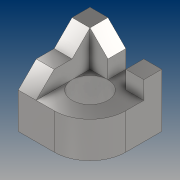
# Autodesk Inventor part: 20
Saved by Autodesk Inventor 2020.2 (Build 242310000, 310)
## iProperties
Created: 2020-09-17
Part Number: 20
Material: 鋼、碳鋼
Document SubType Name: Modeling
Designer: user
Density: 7.85 g/cm^3
Appearance: 半拋光
Mass: 247.275 g
Surface Area: 86.0922 cm^2
Volume: 31.5 cm^3
Author: user
Autodesk Inventor part; units mm, degrees
ref_plane "YZ Plane" through (0, 0, 0) normal (1, 0, 0) x (0, 1, 0)
ref_plane "XZ Plane" through (0, 0, 0) normal (0, 1, 0) x (-1, 0, 0)
ref_plane "XY Plane" through (0, 0, 0) normal (0, 0, 1) x (1, 0, 0)
sketch "草圖1" plane through (0, 0, 0) normal (0, 1, 0) x (-1, 0, 0)
  line L0 (0, 0) -> (-40, 0)
  line L1 (-40, 0) -> (-40, 20)
  arc A0 (-20, 40) -> (-40, 20) centre (-20, 20) ccw
  line L2 (-20, 40) -> (0, 40)
  line L3 (0, 40) -> (0, 0)
  dimension "d0" = 40
  dimension "d1" = 40
  dimension "d2" = 20
  constraints: 8 end point, 3 perpendicular, 2 point on circle, 2 tangent, 1 centre point, 1 horizontal
  measures "d0" distance of L0.start L0.end
  measures "d1" distance of L2.end L0.start
  measures "d2" distance of L2.start L2.end
extrude "擠出1" add sketch "草圖1" along normal blind 20
sketch "草圖2" plane through (0, 0, 0) normal (-1, 0, 0) x (0, 0, 1)
  line L0 (0, 0) -> (0, 20) projected
  line L1 (0, 20) -> (40, 20) projected
  line L2 (40, 20) -> (40, 0) projected
  line L3 (40, 0) -> (0, 0) projected
  line L4 (40, 20) -> (30, 30)
  line L5 (30, 30) -> (20, 30)
  line L6 (20, 30) -> (10, 40)
  line L7 (10, 40) -> (0, 40)
  line L8 (0, 40) -> (0, 20)
  line L9 (40, 20) -> (0, 20)
  dimension "d5" = 10
  dimension "d6" = 10
  dimension "d7" = 10
  dimension "d8" = 10
  constraints: 12 end point, 2 parallel, 2 perpendicular, 1 horizontal
  measures "d5" horizontal distance of L1.end L4.end
  measures "d6" horizontal distance of L1.end L4.end
  measures "d7" horizontal distance of L5.end L6.end
  measures "d8" distance of L6.end L7.end
extrude "擠出2" add sketch "草圖2" against normal blind 10 contours L8 L7 L6 L5 L4 L1
sketch "草圖3" plane through (40, 0, 0) normal (0, 0, -1) x (-1, 0, 0)
  line L0 (30, 40) -> (40, 40) projected
  line L1 (40, 40) -> (40, 0) projected
  line L2 (40, 0) -> (0, 0) projected
  line L3 (0, 0) -> (0, 20) projected
  line L4 (0, 20) -> (30, 20) projected
  line L5 (30, 20) -> (30, 40) projected
  line L6 (30, 40) -> (40, 40) projected
  line L7 (40, 40) -> (40, 0) projected
  line L8 (40, 0) -> (0, 0) projected
  line L9 (0, 0) -> (0, 20) projected
  line L10 (0, 20) -> (30, 20) projected
  line L11 (30, 20) -> (30, 40) projected
  line L12 (30, 40) -> (20, 30)
  line L13 (20, 30) -> (20, 20)
  line L14 (0, 20) -> (10, 20)
  line L15 (10, 20) -> (10, 30)
  line L16 (10, 30) -> (0, 30)
  line L17 (0, 30) -> (0, 20)
  point P0 (10, 20)
  dimension "d11" = 10
  dimension "d12" = 10
  dimension "d13" = 10
  constraints: 12 end point, 2 parallel, 1 horizontal, 1 horizontal alignment, 1 perpendicular, 1 point on line, 1 vertical
  measures "d11" horizontal distance of L0.start L12.end
  measures "d12" distance of L12.end L13.end
  measures "d13" distance of L15.end L16.end
extrude "擠出3" add sketch "草圖3" against normal blind 10 contours L5 L4 L13 L12 | L4 L17 L16 L15
sketch "草圖4" plane through (0, 20, 0) normal (0, 1, 0) x (1, 0, 0)
  arc A0 (20, -40) -> (40, -20) centre (20, -20) ccw projected
  line L0 (20, -40) -> (10, -40) projected
  line L1 (10, -40) -> (0, -40) projected
  line L2 (0, -40) -> (0, 0) projected
  line L3 (0, 0) -> (20, 0) projected
  line L4 (20, 0) -> (30, 0) projected
  line L5 (30, -10) -> (30, 0) projected
  line L6 (40, -10) -> (30, -10) projected
  line L7 (40, 0) -> (40, -10) projected
  line L8 (30, 0) -> (40, 0) projected
  line L9 (40, -10) -> (40, -20) projected
  line L10 (10, -10) -> (10, -40) projected
  line L11 (20, -10) -> (10, -10) projected
  line L12 (20, 0) -> (20, -10) projected
  circle A1 centre (20, -20) radius 10
  line L13 (10, -10) -> (10, -40) projected
  line L14 (20, -10) -> (10, -10) projected
  dimension "d16" = 20
  constraints: 2 tangent, 1 centre point
  measures "d16" diameter of A1
extrude "擠出4" cut sketch "草圖4" against normal blind 36.25 contours A1
